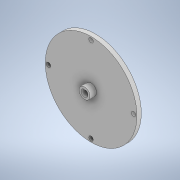
# Autodesk Inventor part: Rotary Motor Coupling
Saved by Autodesk Inventor 2020 (Build 240168000, 168)
## iProperties
Created: 2020-10-19
Part Number: Rotary Motor Coupling
Material: Generic
Document SubType Name: Modeling
Designer: jtri402
Density: 1 g/cm^3
Appearance: Default
Author: jtri402
Autodesk Inventor part; units mm, degrees
ref_plane "YZ Plane" through (0, 0, 0) normal (1, 0, 0) x (0, 1, 0)
ref_plane "XZ Plane" through (0, 0, 0) normal (0, 1, 0) x (-1, 0, 0)
ref_plane "XY Plane" through (0, 0, 0) normal (0, 0, 1) x (1, 0, 0)
sketch "Sketch1" plane through (0, 0, 0) normal (0, 0, 1) x (1, 0, 0)
  point P0 (0, 0)
sketch "Sketch2" plane through (0, 0, 0) normal (0, 0, 1) x (1, 0, 0)
  circle A0 centre (0, 0) radius 210
  dimension "d0" = 420
  constraints: 1 centre point, 1 coincident
  measures "d0" diameter of A0
extrude "Extrusion1" add sketch "Sketch2" along normal blind 20
sketch "Sketch3" plane through (0, 0, 20) normal (0, 0, 1) x (1, 0, 0)
  circle A0 centre (0, 0) radius 25
  circle A1 centre (0, 0) radius 15.875
  dimension "d6" = 50
  dimension "d7" = 31.75
  constraints: 2 centre point, 2 coincident
  measures "d6" diameter of A0
  measures "d7" diameter of A1
extrude "Extrusion2" add sketch "Sketch3" along normal blind 30
extrude "Extrusion3" cut sketch "Sketch3" against normal blind 20 contours A1
sketch "Sketch4" plane through (0, 0, 20) normal (0, 0, 1) x (1, 0, 0)
  circle A0 centre (0, 0) radius 15.875 projected
  circle A1 centre (0, 0) radius 180
  circle A2 centre (0, 195) radius 10
  dimension "d12" = 360
  dimension "d13" = 20
  dimension "d23" = 195
  constraints: 2 centre point, 1 coincident
  measures "d12" diameter of A1
  measures "d13" diameter of A2
  measures "d23" distance of point (0, 0) A2.centre
extrude "Extrusion4" cut sketch "Sketch4" against normal blind 20 contours A2
sketch "Sketch5" plane through (0, 0, 50) normal (0, 0, 1) x (1, 0, 0)
  line L0 (-5, 13.375) -> (5, 13.375)
  line L1 (5, 13.375) -> (5, 18.375)
  line L2 (5, 18.375) -> (-5, 18.375)
  line L3 (-5, 18.375) -> (-5, 13.375)
  circle A0 centre (0, 0) radius 15.875 projected
  line L4 (-5, 13.375) -> (5, 18.375) construction
  line L5 (5, 13.375) -> (-5, 18.375) construction
  point P0 (0, 15.875)
  point P1 (-5, 15.067)
  point P2 (5, 15.067)
  dimension "d19" = 10
  dimension "d20" = 5
  constraints: 12 end point, 2 midpoint, 2 parallel, 1 horizontal, 1 perpendicular, 2 other
  measures "d19" distance of L2.end L1.end
  measures "d20" distance of L1.end L0.end
extrude "Extrusion5" add sketch "Sketch5" against normal blind 30 contours L3 A0 L1 L0 | L3 L2 L1 A0 picked at (-0.5641, 14.1782)
pattern_circular "Circular Pattern1" count 4 over 360 about axis through (0, 0, 0) along (0, 0, 1) of "Extrusion4"
body "Solid1"
